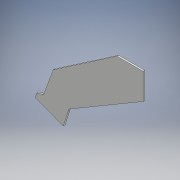
# Autodesk Inventor part: Bras 1
Saved by Autodesk Inventor 2018 (Build 220112000, 112)
## iProperties
Created: 2018-03-19
Part Number: Bras 1
Material: Générique
Document SubType Name: Modeling
Designer: Youri
Density: 1 g/cm^3
Appearance: Par défaut
Author: Youri
Autodesk Inventor part; units mm, degrees
ref_plane "YZ Plane" through (0, 0, 0) normal (1, 0, 0) x (0, 1, 0)
ref_plane "XZ Plane" through (0, 0, 0) normal (0, 1, 0) x (-1, 0, 0)
ref_plane "XY Plane" through (0, 0, 0) normal (0, 0, 1) x (1, 0, 0)
sketch "Esquisse1" plane through (0, 0, 0) normal (0, 1, 0) x (-1, 0, 0)
  line L0 (0, 0) -> (0, 45)
  line L1 (0, 45) -> (45, 45)
  line L2 (0, 0) -> (128, -75.3746)
  line L3 (45, 45) -> (155, -30.3746)
  line L4 (155, -30.3746) -> (171.5194, -75.3746)
  line L5 (128, -75.3746) -> (137.66, -105.3746)
  line L6 (137.66, -105.3746) -> (177.0258, -90.3746)
  line L7 (171.5194, -75.3746) -> (183.1092, -79.0397)
  line L8 (183.1092, -79.0397) -> (186.1095, -86.9134)
  line L9 (186.1095, -86.9134) -> (177.0258, -90.3746)
  dimension "d0" = 45
  dimension "d1" = 45
  dimension "d13" = 128
  dimension "d14" = 110
  dimension "d15" = 30
  dimension "d16" = 45
  constraints: 20 end point, 2 perpendicular, 1 vertical
  measures "d0" distance of L0.end L1.end
  measures "d1" distance of L0.start L0.end
  measures "d13" horizontal distance of L0.start L2.end
  measures "d14" horizontal distance of L1.end L3.end
  measures "d15" vertical distance of L2.end L5.end
  measures "d16" vertical distance of L3.end L4.end
extrude "Extrusion1" add sketch "Esquisse1" along normal blind 3
